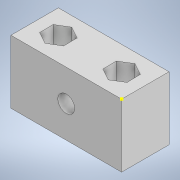
# Autodesk Inventor part: bumper piece 1
Saved by Autodesk Inventor 2022 (Build 260153000, 153)
## iProperties
Created: 2023-01-09
Part Number: bumper piece 1
Material: Generic
Document SubType Name: Modeling
Designer: s143573
Density: 1 g/cm^3
Appearance: Default
Author: s143573
Autodesk Inventor part; units mm, degrees
ref_plane "YZ Plane" through (0, 0, 0) normal (1, 0, 0) x (0, 1, 0)
ref_plane "XZ Plane" through (0, 0, 0) normal (0, 1, 0) x (-1, 0, 0)
ref_plane "XY Plane" through (0, 0, 0) normal (0, 0, 1) x (1, 0, 0)
sketch "Sketch2" plane through (0, 0, 0) normal (0, 1, 0) x (-1, 0, 0)
  line L0 (0, 0) -> (44.45, 0)
  line L1 (44.45, 0) -> (44.45, -19.05)
  line L2 (44.45, -19.05) -> (0, -19.05)
  line L3 (0, -19.05) -> (0, 0)
  dimension "d2" = 19.05
  dimension "d3" = 44.45
  constraints: 8 end point, 2 parallel, 1 horizontal, 1 perpendicular
  measures "d2" distance of L0.end L1.end
  measures "d3" distance of L1.end L2.end
extrude "Extrusion2" add sketch "Sketch2" along normal blind 25.4
sketch "Sketch6" plane through (0, 25.4, 0) normal (0, 1, 0) x (1, 0, 0)
  line L0 (-44.45, 19.05) -> (-44.45, 0) projected
  line L1 (-44.45, 9.525) -> (0, 9.525)
  line L2 (0, 0) -> (0, 19.05) projected
  line L3 (-35.0096, 15.0114) -> (-30.216, 12.3415)
  line L4 (-30.216, 12.3415) -> (-30.1313, 6.8551)
  line L5 (-30.1313, 6.8551) -> (-34.8404, 4.0386)
  line L6 (-34.8404, 4.0386) -> (-39.634, 6.7085)
  line L7 (-39.634, 6.7085) -> (-39.7187, 12.1949)
  line L8 (-39.7187, 12.1949) -> (-35.0096, 15.0114)
  line L9 (-14.3495, 12.1415) -> (-9.6714, 15.0114)
  line L10 (-9.6714, 15.0114) -> (-4.8468, 12.3949)
  line L11 (-4.8468, 12.3949) -> (-4.7005, 6.9085)
  line L12 (-4.7005, 6.9085) -> (-9.3786, 4.0386)
  line L13 (-9.3786, 4.0386) -> (-14.2032, 6.6551)
  line L14 (-14.2032, 6.6551) -> (-14.3495, 12.1415)
  point P0 (-34.925, 9.525)
  point P1 (-9.525, 9.525)
  dimension "d17" = 44.45
  dimension "d18" = 10.9728
  dimension "d19" = 10.9728
  dimension "d20" = 9.525
  dimension "d21" = 9.525
  constraints: 26 end point, 2 midpoint, 2 point on line, 26 other
  measures "d17" distance of L1.start L1.end
  measures "d18" vertical distance of L3.start L5.end
  measures "d19" vertical distance of L9.end L12.end
  measures "d20" distance of L1.start point (-34.925, 9.525)
  measures "d21" distance of L1.end point (-9.525, 9.525)
extrude "Extrusion3" cut sketch "Sketch6" against normal blind 8.382
sketch "Sketch17" plane through (0, 0, -19.05) normal (0, 0, -1) x (-1, 0, 0)
  circle A0 centre (22.225, 12.7) radius 3.3782
  line L0 (44.45, 0) -> (44.45, 25.4) projected
  line L1 (0, 0) -> (44.45, 0) projected
  dimension "d58" = 22.225
  dimension "d59" = 6.7564
  dimension "d68" = 12.7
  constraints: 1 centre point
  measures "d58" distance from line of L0 A0.centre
  measures "d59" diameter of A0
  measures "d68" distance from line of L1 A0.centre
extrude "Extrusion11" cut sketch "Sketch17" against normal blind 25.4
sketch "Sketch19" plane through (0, 25.4, 0) normal (0, 1, 0) x (1, 0, 0)
  point P0 (0, 0)
sketch "Sketch20" plane through (0, 25.4, 0) normal (0, 1, 0) x (1, 0, 0)
  line L0 (-4.7005, 6.9085) -> (-9.3786, 4.0386) projected
  line L1 (-9.3786, 4.0386) -> (-14.2032, 6.6551) projected
  line L2 (-14.2032, 6.6551) -> (-14.3495, 12.1415) projected
  line L3 (-14.3495, 12.1415) -> (-9.6714, 15.0114) projected
  line L4 (-9.6714, 15.0114) -> (-4.8468, 12.3949) projected
  line L5 (-4.8468, 12.3949) -> (-4.7005, 6.9085) projected
  line L6 (-14.3495, 12.1415) -> (-9.6714, 15.0114) projected
  line L7 (-14.2032, 6.6551) -> (-14.3495, 12.1415) projected
  line L8 (-9.3786, 4.0386) -> (-14.2032, 6.6551) projected
  line L9 (-4.7005, 6.9085) -> (-9.3786, 4.0386) projected
  line L10 (-4.8468, 12.3949) -> (-4.7005, 6.9085) projected
  line L11 (-9.6714, 15.0114) -> (-4.8468, 12.3949) projected
  line L12 (-30.1313, 6.8551) -> (-34.8404, 4.0386) projected
  line L13 (-30.216, 12.3415) -> (-30.1313, 6.8551) projected
  line L14 (-35.0096, 15.0114) -> (-30.216, 12.3415) projected
  line L15 (-39.7187, 12.1949) -> (-35.0096, 15.0114) projected
  line L16 (-39.634, 6.7085) -> (-39.7187, 12.1949) projected
  line L17 (-34.8404, 4.0386) -> (-39.634, 6.7085) projected
  line L18 (-4.7005, 6.9085) -> (-9.3786, 4.0386) projected
  line L19 (-9.3786, 4.0386) -> (-9.6714, 15.0114)
  line L20 (-4.8468, 12.3949) -> (-4.7005, 6.9085) projected
  line L21 (-4.7736, 9.6517) -> (-14.2764, 9.3983)
  line L22 (-14.2032, 6.6551) -> (-14.3495, 12.1415) projected
  circle A0 centre (-9.525, 9.525) radius 3.3782
  line L23 (-34.8404, 4.0386) -> (-35.0096, 15.0114)
  line L24 (-39.634, 6.7085) -> (-39.7187, 12.1949) projected
  line L25 (-39.6764, 9.4517) -> (-30.1736, 9.5983)
  line L26 (-30.216, 12.3415) -> (-30.1313, 6.8551) projected
  circle A1 centre (-34.925, 9.525) radius 3.3782
  point P0 (0, 0)
  dimension "d64" = 6.7564
  dimension "d65" = 6.7564
  constraints: 8 end point, 6 midpoint, 2 centre point, 2 point on line
  measures "d64" diameter of A0
  measures "d65" diameter of A1
extrude "Extrusion12" cut sketch "Sketch20" against normal through all contours A0 L21 L19 | L19 L21 A0 | L21 L19 A0 | L21 A0 L19 | A1 L25 L23 | L23 L25 A1 | L25 L23 A1 | L25 A1 L23
sketch "Sketch21" plane through (0, 25.4, 0) normal (0, 1, 0) x (1, 0, 0)
  point P0 (0, 0)
body "Solid2"
